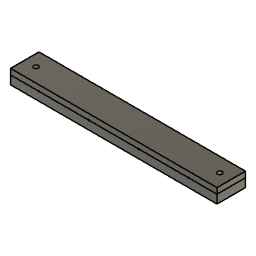
Alignment Clip (Autodesk Fusion 360 design; units mm, degrees)
Autodesk Fusion 360 part; units mm, degrees
note: some values were not read from the file. Set by a fixed rule: which sketch regions a step uses.
sketch "sketch 226" plane through (0, 0, 0) normal (0, 1, 0) x (1, 0, 0)
  line L0 (0, 0) -> (145, 0)
  line L1 (145, 0) -> (145, 6)
  line L2 (145, 6) -> (0, 6)
  line L3 (0, 6) -> (0, 0)
  circle A0 centre (20, 0) radius 0.45
  circle A1 centre (55, 0) radius 0.45
  circle A2 centre (125, 0) radius 0.45
  circle A3 centre (90, 0) radius 0.45
  line L4 (0, 0) -> (145, 0)
  line L5 (145, 0) -> (145, -6)
  line L6 (145, -6) -> (0, -6)
  line L7 (0, -6) -> (0, 0)
  constraint horizontal L0
  constraint vertical L1
  constraint horizontal L2
  constraint vertical L3
  constraint coincident L0.start L3.end
  constraint coincident L0 A0.centre
  constraint coincident L0 A1.centre
  constraint coincident L0 A2.centre
  constraint coincident L0 A3.centre
  constraint horizontal L4
  constraint vertical L5
  constraint horizontal L6
  constraint vertical L7
extrude "Extrude1" add sketch "sketch 226" along normal blind 20 contours L0 A0 A1 A2 A3 L4 L5 L6 L7 makes body 1
extrude "Extrude2" add sketch "sketch 226" along normal blind 20 separate body contours L0 L1 L2 L3 A0 A1 A2 A3 L4 makes body 2
sketch "Sketch1" plane through (0, 0, -6) normal (0, 0, -1) x (1, 0, 0)
  line L0 (145, 0) -> (0, 0)
  line L1 (0, 0) -> (0, -20)
  line L2 (0, -20) -> (145, -20)
  line L3 (145, -20) -> (145, 0)
  line L4 (0, 0) -> (8, 0)
  line L5 (8, 0) -> (8, -10)
  line L6 (8, -10) -> (0, -10)
  line L7 (0, -10) -> (0, 0)
  line L8 (145, 0) -> (137, 0)
  line L9 (137, 0) -> (137, -10)
  line L10 (137, -10) -> (145, -10)
  line L11 (145, -10) -> (145, 0)
  circle A0 centre (8, -10) radius 2
  circle A1 centre (8, -10) radius 1.65
  circle A2 centre (137, -10) radius 2
  circle A3 centre (137, -10) radius 1.65
  dimension "d5" = 8
  dimension "d6" = 10
  dimension "d7" = 8
  dimension "d8" = 10
  dimension "d9" = 4
  dimension "d10" = 3.3
  dimension "d11" = 4
  dimension "d12" = 3.3
  constraint horizontal L4
  constraint vertical L5
  constraint horizontal L6
  constraint vertical L7
  constraint coincident L0.end L1.start
  constraint horizontal L8
  constraint vertical L9
  constraint horizontal L10
  constraint vertical L11
  constraint coincident L0.start L3.end
  constraint coincident L5.end L6.start
  constraint concentric A0 A1
  constraint coincident L9.end L10.start
  measures "d5" distance of L0.end L4.end
  measures "d6" distance of L0.end L6.end
  measures "d7" distance of L0.start L8.end
  measures "d8" distance of L0.start L10.end
  measures "d9" diameter of A0
  measures "d10" diameter of A1
  measures "d11" diameter of A2
  measures "d12" diameter of A3
extrude "Extrude3" cut sketch "Sketch1" against normal blind 12 contours L9 L10 A3 | L9 L10 A3 | L5 L6 A1 | L5 L6 A1 bodies 1 2
extrude "Extrude4" cut sketch "Sketch1" against normal blind 5 contours L9 L10 A2 A3 | L9 L10 A2 A3 | L5 L6 A0 A1 | L5 L6 A0 A1 bodies 2
extrude "Extrude5" cut 1 faces at (51.3535, 2.912, 6) along direction (0, 0, -1) blind 2 on bodies 1 bodies 1
